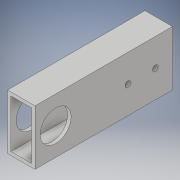
# Autodesk Inventor part: Gearbox Shaft Stabilizer
Saved by Autodesk Inventor 2018 (Build 220112000, 112)
## iProperties
Created: 2019-03-02
Part Number: Gearbox Shaft Stabilizer
Material: Generic
Document SubType Name: Modeling
Designer: s-4009421
Density: 1 g/cm^3
Appearance: Default
Author: s-4009421
Autodesk Inventor part; units mm, degrees
ref_plane "YZ Plane" through (0, 0, 0) normal (1, 0, 0) x (0, 1, 0)
ref_plane "XZ Plane" through (0, 0, 0) normal (0, 1, 0) x (-1, 0, 0)
ref_plane "XY Plane" through (0, 0, 0) normal (0, 0, 1) x (1, 0, 0)
sketch "Sketch1" plane through (0, 0, 0) normal (0, 0, 1) x (1, 0, 0)
  line L0 (-6.6707, 4.0865) -> (18.7293, 4.0865)
  line L1 (18.7293, 4.0865) -> (18.7293, -46.7135)
  line L2 (18.7293, -46.7135) -> (-6.6707, -46.7135)
  line L3 (-6.6707, -46.7135) -> (-6.6707, 4.0865)
  line L4 (15.5543, 0.9115) -> (-3.4957, 0.9115)
  line L5 (-3.4957, 0.9115) -> (-3.4957, -43.5385)
  line L6 (-3.4957, -43.5385) -> (15.5543, -43.5385)
  line L7 (15.5543, -43.5385) -> (15.5543, 0.9115)
  point P0 (0, 0)
  dimension "d0" = 25.4
  dimension "d1" = 50.8
  dimension "d2" = 3.175
  constraints: 16 end point, 4 parallel, 2 perpendicular, 1 horizontal, 3 other
  measures "d0" distance of L1.end L2.end
  measures "d1" distance of L0.end L1.end
  measures "d2" distance between parallel lines of L0 L4
extrude "Extrusion1" add sketch "Sketch1" along normal blind 127
sketch "Sketch2" plane through (18.7293, -46.7135, 0) normal (1, 0, 0) x (0, 0, -1)
  line L0 (0, 47.625) -> (0, 3.175) projected
  line L1 (0, 25.4) -> (-107.95, 25.4)
  circle A0 centre (-107.95, 25.4) radius 14.2875
  point P0 (0, 46.7135)
  dimension "d5" = 107.95
  dimension "d6" = 28.575
  constraints: 2 end point, 1 centre point, 1 coincident, 1 horizontal, 1 midpoint
  measures "d5" distance of L1.start L1.end
  measures "d6" diameter of A0
extrude "Extrusion2" cut sketch "Sketch2" against normal blind 101.6
sketch "Sketch3" plane through (18.7293, -46.7135, 0) normal (1, 0, 0) x (0, 0, -1)
  line L0 (0, 47.625) -> (0, 3.175) projected
  line L1 (0, 25.4) -> (-15.875, 25.4)
  line L2 (-15.875, 25.4) -> (-41.275, 25.4)
  circle A0 centre (-15.875, 25.4) radius 2.5797
  circle A1 centre (-41.275, 25.4) radius 2.5797
  point P0 (0, 46.7135)
  dimension "d9" = 15.875
  dimension "d10" = 25.4
  dimension "d11" = 5.1594
  dimension "d12" = 5.1594
  constraints: 4 end point, 2 centre point, 2 coincident, 1 horizontal, 1 midpoint, 1 point on line
  measures "d9" distance of L1.start L1.end
  measures "d10" distance of L1.end L2.end
  measures "d11" diameter of A0
  measures "d12" diameter of A1
extrude "Extrusion3" cut sketch "Sketch3" against normal blind 101.6
body "Solid1"
